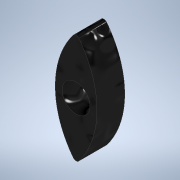
# Autodesk Inventor part: LongCarriageGuide
Saved by Autodesk Inventor 2020.2 (Build 242310000, 310)
## iProperties
Created: 2020-03-12
Part Number: LongCarriageGuide
Material: Generic
Document SubType Name: Modeling
Designer: elmar
Density: 1 g/cm^3
Appearance: Black
Author: elmar
Autodesk Inventor part; units mm, degrees
ref_plane "YZ Plane" through (0, 0, 0) normal (1, 0, 0) x (0, 1, 0)
ref_plane "XZ Plane" through (0, 0, 0) normal (0, 1, 0) x (-1, 0, 0)
ref_plane "XY Plane" through (0, 0, 0) normal (0, 0, 1) x (1, 0, 0)
sketch "Sketch1" plane through (0, 0, 0) normal (0, 0, 1) x (1, 0, 0)
  circle A0 centre (0, 0) radius 4
  circle A1 centre (0, 0) radius 6
  arc A2 (0, 16.2481) -> (0, -16.2481) centre (19, 0) ccw
  arc A3 (0, -16.2481) -> (0, 16.2481) centre (-19, 0) ccw
  line L0 (-26.6, 0) -> (26.6, 0) projected
  line L1 (0, -23.1325) -> (0, 25.0583) projected
  line L2 (0, 16.2481) -> (-1.2304, 17.6868)
  line L3 (0, 16.2481) -> (1.6469, 18.1739)
  dimension "d0" = 12
  dimension "d1" = 8
  dimension "d2" = 25
  dimension "d6" = 81.072
  constraints: 4 centre point, 4 end point, 4 point on circle, 4 tangent, 3 point on line, 2 coincident
  measures "d0" diameter of A1
  measures "d1" diameter of A0
  measures "d2" radius of A2
  measures "d6" angle of L3 L2
extrude "Extrusion1" add sketch "Sketch1" along normal blind 8 contours L0 A1 L1 A0 | A0 L1 A1 L0 | A0 L0 A1 L1 | L1 A1 L0 A0 | A3 L1 A1 | A1 L1 A3 | A1 A2 L1 | L1 A2 A1
fillet "Fillet1" radius 1 2 edges at (0, 16.2481, 4) (0, -16.2481, 4)
body "Solid1"
